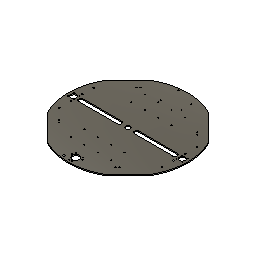
Baseplate-3mm (Autodesk Fusion 360 design; units mm, degrees)
Autodesk Fusion 360 part; units mm, degrees
sketch "Skizze1" plane through (0, 0, 0) normal (0, 0, 1) x (1, 0, 0)
  line L0 (0, 0) -> (-150, 0) construction
  line L1 (0, 0) -> (-24, 0) construction
  line L2 (-14, 0) -> (-130, 0) construction
  line L3 (0, 0) -> (95.4594, 95.4594) construction
  line L4 (0, 0) -> (-95.4594, 95.4594) construction
  line L5 (0, 0) -> (95.4594, -95.4594) construction
  line L6 (0, 0) -> (-95.4594, -95.4594) construction
  line L7 (-150, -16) -> (-142, -16) construction
  circle A0 centre (-142, -16) radius 2.1
  line L8 (-142, -16) -> (-142, -48) construction
  circle A1 centre (-142, -48) radius 2.1
  line L9 (-111.7229, 111.7229) -> (-78.1, 145.3458)
  line L10 (-111.7229, 111.7229) -> (-145.3458, 78.1)
  line L11 (95.4594, 95.4594) -> (111.7229, 111.7229) construction
  line L12 (111.7229, 111.7229) -> (145.3458, 78.1)
  line L13 (111.7229, 111.7229) -> (78.1, 145.3458)
  arc A2 (78.1, 145.3458) -> (-78.1, 145.3458) centre (0, 0) ccw
  line L14 (111.7229, -111.7229) -> (145.3458, -78.1)
  line L15 (111.7229, -111.7229) -> (78.1, -145.3458)
  arc A3 (145.3458, -78.1) -> (145.3458, 78.1) centre (0, 0) ccw
  line L16 (-111.7229, -111.7229) -> (-78.1, -145.3458)
  line L17 (-111.7229, -111.7229) -> (-145.3458, -78.1)
  arc A4 (-145.3458, 78.1) -> (-145.3458, -78.1) centre (0, 0) ccw
  arc A5 (-78.1, -145.3458) -> (78.1, -145.3458) centre (0, 0) ccw
  line L18 (-150, 16) -> (-142, 16) construction
  circle A6 centre (-142, 16) radius 2.1
  line L19 (-142, 16) -> (-142, 48) construction
  circle A7 centre (-142, 48) radius 2.1
  arc A8 (-24, -6.25) -> (-24, 6.25) centre (-24, 0) ccw
  arc A9 (-130, 6.25) -> (-130, -6.25) centre (-130, 0) ccw
  circle A10 centre (142, 48) radius 2.1
  circle A11 centre (142, -16) radius 2.1
  circle A12 centre (142, 16) radius 2.1
  line L20 (150, 0) -> (150, -16) construction
  line L21 (150, 0) -> (150, 16) construction
  line L22 (150, 16) -> (142, 16) construction
  line L23 (142, 16) -> (142, 48) construction
  line L24 (150, 0) -> (0, 0) construction
  line L25 (-0.0142, -0.0056) -> (23.9858, -0.0056) construction
  line L26 (14, -0.0076) -> (129.9927, -0.1231) construction
  arc A13 (129.9858, -6.3731) -> (129.9996, 6.1269) centre (129.9927, -0.1231) ccw
  line L27 (150, -16) -> (142, -16) construction
  line L28 (142, -16) -> (142, -48) construction
  circle A14 centre (142, -48) radius 2.1
  circle A15 centre (0, 0) radius 6.5
  line L29 (0, 0) -> (0, -144) construction
  circle A16 centre (0, -144) radius 10
  line L30 (0, -144) -> (-14, -144) construction
  line L31 (0, -144) -> (-10.6066, -133.3934) construction
  circle A17 centre (-10.6066, -133.3934) radius 1.5
  line L32 (0, -144) -> (-3.8823, -158.4889) construction
  circle A18 centre (-3.8823, -158.4889) radius 1.5
  line L33 (0, -144) -> (3.6235, -157.523) construction
  circle A19 centre (3.6235, -157.523) radius 1.5
  line L34 (0, -144) -> (9.8995, -134.1005) construction
  circle A20 centre (9.8995, -134.1005) radius 1.5
  line L35 (0, -144) -> (14.4889, -140.1177) construction
  circle A21 centre (14.4889, -140.1177) radius 1.5
  line L36 (0, 0) -> (0, -65) construction
  line L37 (0, -65) -> (18.5, -65) construction
  line L38 (18.5, -65) -> (18.5, -101.9) construction
  line L39 (18.5, -101.9) -> (-18.5, -101.9) construction
  line L40 (-18.5, -101.9) -> (-18.5, -65) construction
  circle A22 centre (-18.5, -65) radius 1.35
  circle A23 centre (-18.5, -101.9) radius 1.35
  circle A24 centre (18.5, -101.9) radius 1.35
  circle A25 centre (18.5, -65) radius 1.35
  line L41 (0, 0) -> (0, 65) construction
  line L42 (0, 65) -> (18.5, 65) construction
  line L43 (18.5, 65) -> (18.5, 101.9) construction
  line L44 (18.5, 101.9) -> (-18.5, 101.9) construction
  line L45 (-18.5, 101.9) -> (-18.5, 65) construction
  circle A26 centre (-18.5, 65) radius 1.35
  circle A27 centre (18.5, 65) radius 1.35
  circle A28 centre (18.5, 101.9) radius 1.35
  circle A29 centre (-18.5, 101.9) radius 1.35
  line L46 (18.5, -65) -> (55.4, -65) construction
  line L47 (18.5, -101.9) -> (55.4, -101.9) construction
  line L48 (-18.5, -65) -> (-55.4, -65) construction
  line L49 (-18.5, -101.9) -> (-55.4, -101.9) construction
  circle A30 centre (55.4, -65) radius 1.35
  circle A31 centre (55.4, -101.9) radius 1.35
  circle A32 centre (-55.4, -65) radius 1.35
  circle A33 centre (-55.4, -101.9) radius 1.35
  line L50 (18.5, 101.9) -> (55.4, 101.9) construction
  line L51 (18.5, 65) -> (55.4, 65) construction
  line L52 (-18.5, 65) -> (-55.4, 65) construction
  line L53 (-18.5, 101.9) -> (-55.4, 101.9) construction
  circle A34 centre (-55.4, 101.9) radius 1.35
  circle A35 centre (-55.4, 65) radius 1.35
  circle A36 centre (55.4, 65) radius 1.35
  circle A37 centre (55.4, 101.9) radius 1.35
  line L54 (-150, 16) -> (-150, 0) construction
  line L55 (-150, 0) -> (-150, -16) construction
  circle A38 centre (150, 0) radius 8.05
  circle A39 centre (-150, 0) radius 8.05
  line L56 (-150, 0) -> (-150, 8) construction
  line L57 (-150, 8) -> (-142, 8) construction
  line L58 (-142, 8) -> (-142, -8) construction
  line L59 (-142, -8) -> (-158, -8) construction
  line L60 (-158, -8) -> (-158, 8) construction
  circle A40 centre (-158, 8) radius 1.1
  circle A41 centre (-142, 8) radius 1.1
  circle A42 centre (-142, -8) radius 1.1
  circle A43 centre (-158, -8) radius 1.1
  line L61 (150, 0) -> (150, 8.0016) construction
  line L62 (150, 8.0016) -> (142, 8.0016) construction
  line L63 (142, 8.0016) -> (142, -7.9984) construction
  line L64 (142, -7.9984) -> (158, -7.9984) construction
  line L65 (158, -7.9984) -> (158, 8.0016) construction
  circle A44 centre (158, -7.9984) radius 1.1
  circle A45 centre (142, -7.9984) radius 1.1
  circle A46 centre (142, 8.0016) radius 1.1
  circle A47 centre (158, 8.0016) radius 1.1
  line L66 (0, 65) -> (0, 110) construction
  line L67 (0, 110) -> (-20, 110) construction
  circle A48 centre (-20, 110) radius 1.35
  line L68 (-20, 110) -> (32.1, 110.0005) construction
  line L69 (32.1, 110.0005) -> (32.1, 115.1005) construction
  circle A49 centre (32.1, 115.1005) radius 1.35
  line L70 (32.1, 115.1005) -> (32.1, 143.0005) construction
  circle A50 centre (32.1, 143.0005) radius 1.35
  line L71 (32.1, 143.0005) -> (32.1, 158.2005) construction
  line L72 (32.1, 158.2005) -> (-18.7, 158.2005) construction
  circle A51 centre (-18.7, 158.2005) radius 1.35
  line L73 (-130, 6.25) -> (-24, 6.25)
  line L74 (23.9879, 6.2444) -> (129.9996, 6.1269)
  line L75 (23.9858, -0.0056) -> (23.9858, -6.2556) construction
  line L76 (129.9858, -6.3731) -> (23.9858, -6.2556)
  line L77 (23.9858, -0.0056) -> (23.9858, 6.0001) construction
  line L78 (-24, 0) -> (-24, -6.25) construction
  line L79 (-24, -6.25) -> (-130, -6.25)
  arc A52 (23.9879, 6.2444) -> (23.9858, -6.2556) centre (23.9858, -0.0056) ccw
  line L80 (0, -144) -> (-13.523, -140.3765) construction
  line L81 (0, -144) -> (-12.5631, -144) construction
  circle A53 centre (-13.523, -140.3765) radius 1.5
  line L82 (-95.4594, -95.4594) -> (-107.1267, -83.7922) construction
  line L83 (-107.1267, -83.7922) -> (-112.8542, -78.0646) construction
  circle A54 centre (-107.1267, -83.7922) radius 1.5
  circle A55 centre (-112.8542, -78.0646) radius 1.5
  line L84 (-95.4594, 95.4594) -> (-83.7922, 107.1267) construction
  line L85 (-83.7922, 107.1267) -> (-78.0646, 112.8542) construction
  line L86 (-83.7922, 107.1267) -> (-69.8987, 107.1267) construction
  circle A56 centre (-83.7922, 107.1267) radius 1.5
  circle A57 centre (-78.0646, 112.8542) radius 1.5
  line L87 (95.4594, 95.4594) -> (107.1267, 83.7922) construction
  line L88 (107.1267, 83.7922) -> (112.8542, 78.0646) construction
  circle A58 centre (107.1267, 83.7922) radius 1.5
  circle A59 centre (112.8542, 78.0646) radius 1.5
  line L89 (95.4594, -95.4594) -> (83.7922, -107.1267) construction
  line L90 (83.7922, -107.1267) -> (78.0646, -112.8542) construction
  circle A60 centre (83.7922, -107.1267) radius 1.5
  circle A61 centre (78.0646, -112.8542) radius 1.5
  line L91 (0, -144) -> (-20.7846, -156) construction
  circle A62 centre (-20.7846, -156) radius 2.65
  dimension "d144" = 4.2
  dimension "d148" = 4.2
  dimension "d185" = 4.2
  dimension "d187" = 4.2
  dimension "d306" = 12.5
  dimension "d309" = 12.5
  dimension "d333" = 4.2
  dimension "d335" = 4.2
  dimension "d338" = 4.2
  dimension "d371" = 12.5
  dimension "d383" = 4.2
  dimension "d386" = 13
  dimension "d390" = 20
  dimension "d400" = 3
  dimension "d402" = 3
  dimension "d405" = 3
  dimension "d408" = 3
  dimension "d411" = 3
  dimension "d419" = 2.7
  dimension "d420" = 2.7
  dimension "d421" = 2.7
  dimension "d422" = 2.7
  dimension "d428" = 2.7
  dimension "d429" = 2.7
  dimension "d430" = 2.7
  dimension "d431" = 2.7
  dimension "d438" = 2.7
  dimension "d439" = 2.7
  dimension "d440" = 2.7
  dimension "d441" = 2.7
  dimension "d446" = 2.7
  dimension "d447" = 2.7
  dimension "d448" = 2.7
  dimension "d449" = 2.7
  dimension "d456" = 16.1
  dimension "d457" = 16.1
  dimension "d463" = 2.2
  dimension "d464" = 2.2
  dimension "d465" = 2.2
  dimension "d466" = 2.2
  dimension "d473" = 2.2
  dimension "d474" = 2.2
  dimension "d475" = 2.2
  dimension "d476" = 2.2
  dimension "d483" = 45
  dimension "d484" = 20
  dimension "d485" = 2.7
  dimension "d488" = 2.7
  dimension "d490" = 5.1
  dimension "d491" = 27.9
  dimension "d492" = 52.1
  dimension "d493" = 2.7
  dimension "d494" = 15.2
  dimension "d495" = 50.8
  dimension "d497" = 2.7
  dimension "d505" = 144
  dimension "d506" = 135
  dimension "d507" = 45
  dimension "d508" = 165
  dimension "d509" = 105
  dimension "d510" = 75
  dimension "d511" = 14
  dimension "d512" = 15
  dimension "d513" = 14
  dimension "d514" = 15
  dimension "d515" = 14
  dimension "d516" = 15
  dimension "d522" = 106
  dimension "d526" = 106
  dimension "d527" = 12.5
  dimension "d530" = 150
  dimension "d531" = 150
  dimension "d532" = 8
  dimension "d533" = 16
  dimension "d534" = 16
  dimension "d535" = 16
  dimension "d536" = 16
  dimension "d537" = 16
  dimension "d538" = 8
  dimension "d539" = 32
  dimension "d540" = 32
  dimension "d541" = 8
  dimension "d542" = 32
  dimension "d543" = 8
  dimension "d544" = 16
  dimension "d545" = 16
  dimension "d546" = 16
  dimension "d547" = 16
  dimension "d548" = 8
  dimension "d549" = 16
  dimension "d550" = 8
  dimension "d551" = 32
  dimension "d552" = 135
  dimension "d553" = 135
  dimension "d554" = 135
  dimension "d555" = 135
  dimension "d564" = 36.9
  dimension "d565" = 36.9
  dimension "d566" = 36.9
  dimension "d567" = 37
  dimension "d568" = 18.5
  dimension "d569" = 36.9
  dimension "d570" = 36.9
  dimension "d571" = 36.9
  dimension "d572" = 65
  dimension "d575" = 47.55
  dimension "d576" = 47.55
  dimension "d577" = 165
  dimension "d578" = 47.55
  dimension "d579" = 47.55
  dimension "d580" = 165
  dimension "d581" = 47.55
  dimension "d582" = 47.55
  dimension "d583" = 165
  dimension "d584" = 47.55
  dimension "d585" = 47.55
  dimension "d586" = 165
  dimension "d589" = 15
  dimension "d590" = 14
  dimension "d591" = 3
  dimension "d594" = 36.9
  dimension "d595" = 36.9
  dimension "d596" = 36.9
  dimension "d597" = 37
  dimension "d598" = 18.5
  dimension "d599" = 36.9
  dimension "d600" = 36.9
  dimension "d601" = 36.9
  dimension "d604" = 16.5
  dimension "d605" = 8.1
  dimension "d606" = 3
  dimension "d607" = 3
  dimension "d608" = 16.5
  dimension "d609" = 45
  dimension "d610" = 8.1
  dimension "d611" = 3
  dimension "d612" = 3
  dimension "d613" = 16.5
  dimension "d614" = 8.1
  dimension "d615" = 3
  dimension "d616" = 3
  dimension "d617" = 16.5
  dimension "d618" = 8.1
  dimension "d619" = 3
  dimension "d620" = 3
  dimension "d623" = 24
  dimension "d624" = 24
  dimension "d631" = 24
  dimension "d632" = 45
  dimension "d633" = 5.3
  constraint coincident L0.start L1.start
  constraint parallel L0 L1
  constraint parallel L0 L2
  constraint coincident L7.end A0.centre
  constraint perpendicular L7 L8
  constraint coincident L8.end A1.centre
  constraint concentric A2 A4
  constraint concentric A3 A4
  constraint concentric A4 A5
  constraint coincident L18.end A6.centre
  constraint perpendicular L18 L19
  constraint coincident L19.end A7.centre
  constraint coincident L1.end A8.centre
  constraint coincident L2.end A9.centre
  constraint perpendicular L21 L22
  constraint coincident A12.centre L22.end
  constraint perpendicular L22 L23
  constraint coincident A10.centre L23.end
  constraint perpendicular L21 L24
  constraint parallel L24 L25
  constraint coincident L26.end A13.centre
  constraint perpendicular L20 L24
  constraint coincident A11.centre L27.end
  constraint perpendicular L27 L28
  constraint coincident L28.end A14.centre
  constraint concentric A5 A15
  constraint vertical L29
  constraint coincident L29.end A16.centre
  constraint perpendicular L29 L30
  constraint coincident L31.end A17.centre
  constraint coincident L32.end A18.centre
  constraint coincident L33.end A19.centre
  constraint coincident L34.end A20.centre
  constraint coincident L35.end A21.centre
  constraint perpendicular L25 L36
  constraint perpendicular L29 L37
  constraint perpendicular L37 L38
  constraint perpendicular L38 L39
  constraint perpendicular L39 L40
  constraint coincident L40.end A22.centre
  constraint coincident L39.end L40.start
  constraint coincident L38.end L39.start
  constraint coincident L37.end L38.start
  constraint perpendicular L24 L41
  constraint perpendicular L41 L42
  constraint perpendicular L42 L43
  constraint perpendicular L43 L44
  constraint perpendicular L44 L45
  constraint coincident L45.end A26.centre
  constraint coincident L42.end L43.start
  constraint coincident L43.end L44.start
  constraint coincident L44.end L45.start
  constraint perpendicular L38 L46
  constraint perpendicular L38 L47
  constraint perpendicular L40 L48
  constraint perpendicular L40 L49
  constraint coincident L46.end A30.centre
  constraint coincident L47.end A31.centre
  constraint coincident L48.end A32.centre
  constraint coincident L49.end A33.centre
  constraint perpendicular L43 L50
  constraint perpendicular L43 L51
  constraint perpendicular L45 L52
  constraint perpendicular L45 L53
  constraint coincident L53.end A34.centre
  constraint coincident L52.end A35.centre
  constraint coincident L51.end A36.centre
  constraint coincident L50.end A37.centre
  constraint perpendicular L0 L54
  constraint perpendicular L7 L55
  constraint perpendicular L18 L54
  constraint perpendicular L0 L55
  constraint perpendicular L20 L27
  constraint coincident L20.start L21.start
  constraint coincident L0.end L54.end
  constraint perpendicular L0 L56
  constraint perpendicular L56 L57
  constraint perpendicular L0 L58
  constraint perpendicular L55 L59
  constraint perpendicular L59 L60
  constraint coincident L60.end A40.centre
  constraint coincident L57.end L58.start
  constraint coincident L58.end L59.start
  constraint coincident L59.end L60.start
  constraint perpendicular L24 L61
  constraint perpendicular L61 L62
  constraint perpendicular L62 L63
  constraint perpendicular L20 L64
  constraint perpendicular L64 L65
  constraint coincident L64.end L65.start
  constraint coincident L63.end L64.start
  constraint coincident L62.end L63.start
  constraint coincident L65.end A47.centre
  constraint perpendicular L44 L66
  constraint perpendicular L66 L67
  constraint coincident L67.end A48.centre
  constraint perpendicular L68 L69
  constraint coincident L69.end A49.centre
  constraint vertical L41
  constraint vertical L70
  constraint coincident L70.end A50.centre
  constraint parallel L70 L71
  constraint perpendicular L71 L72
  constraint coincident L72.end A51.centre
  constraint horizontal L73
  constraint tangent A13 L74
  constraint perpendicular L24 L75
  constraint perpendicular L24 L77
  constraint perpendicular L1 L78
  constraint coincident L25.end L75.start
  constraint horizontal L0
  constraint horizontal L81
  constraint coincident L80.end A53.centre
  constraint perpendicular L6 L82
  constraint parallel L82 L83
  constraint coincident L82.end L83.start
  constraint coincident L83.end A55.centre
  constraint perpendicular L4 L84
  constraint horizontal L86
  constraint coincident L84.end L85.start
  constraint coincident L85.end A57.centre
  constraint perpendicular L3 L87
  constraint perpendicular L3 L88
  constraint coincident L87.end L88.start
  constraint coincident L88.end A59.centre
  constraint perpendicular L5 L89
  constraint parallel L89 L90
  constraint coincident L89.end L90.start
  constraint coincident L90.end A61.centre
  constraint tangent A13 L76
  constraint tangent A9 L73
  constraint tangent A8 L73
  constraint tangent A9 L79
  constraint coincident L91.end A62.centre
  measures "d144" diameter of A0
  measures "d148" diameter of A1
  measures "d185" diameter of A6
  measures "d187" diameter of A7
  measures "d306" diameter of A8
  measures "d309" diameter of A9
  measures "d333" diameter of A12
  measures "d335" diameter of A10
  measures "d338" diameter of A11
  measures "d371" diameter of A13
  measures "d383" diameter of A14
  measures "d386" diameter of A15
  measures "d390" diameter of A16
  measures "d400" diameter of A17
  measures "d402" diameter of A18
  measures "d405" diameter of A19
  measures "d408" diameter of A20
  measures "d411" diameter of A21
  measures "d419" diameter of A22
  measures "d420" diameter of A23
  measures "d421" diameter of A24
  measures "d422" diameter of A25
  measures "d428" diameter of A26
  measures "d429" diameter of A27
  measures "d430" diameter of A28
  measures "d431" diameter of A29
  measures "d438" diameter of A30
  measures "d439" diameter of A31
  measures "d440" diameter of A32
  measures "d441" diameter of A33
  measures "d446" diameter of A34
  measures "d447" diameter of A35
  measures "d448" diameter of A36
  measures "d449" diameter of A37
  measures "d456" diameter of A38
  measures "d457" diameter of A39
  measures "d463" diameter of A40
  measures "d464" diameter of A41
  measures "d465" diameter of A42
  measures "d466" diameter of A43
  measures "d473" diameter of A44
  measures "d474" diameter of A45
  measures "d475" diameter of A46
  measures "d476" diameter of A47
  measures "d483" distance of L41.end L66.end
  measures "d484" distance of L66.end L67.end
  measures "d485" diameter of A48
  measures "d488" diameter of A49
  measures "d490" vertical distance of L68.end L69.end
  measures "d491" distance of L69.end L70.end
  measures "d492" horizontal distance of L67.end L68.end
  measures "d493" diameter of A50
  measures "d494" distance of L70.end L71.end
  measures "d495" distance of L71.end L72.end
  measures "d497" diameter of A51
  measures "d505" distance of L0.start L29.end
  measures "d506" angle of L30 L34
  measures "d507" angle of L30 L31
  measures "d508" angle of L30 L35
  measures "d509" angle of L30 L33
  measures "d510" angle of L30 L32
  measures "d511" distance of L29.end L34.end
  measures "d512" distance of L29.end L35.end
  measures "d513" distance of L29.end L33.end
  measures "d514" distance of L29.end L32.end
  measures "d515" distance of L29.end L30.end
  measures "d516" distance of L29.end L31.end
  measures "d522" distance of A13.start L75.end
  measures "d526" distance of A9.end A8.start
  measures "d527" diameter of A52
  measures "d530" distance of L0.start L0.end
  measures "d531" distance of L0.start L20.start
  measures "d532" distance of L56.end L57.end
  measures "d533" distance of L57.end L58.end
  measures "d534" distance of L58.end L59.end
  measures "d535" distance of L59.end L60.end
  measures "d536" distance of L0.end L18.start
  measures "d537" distance of L0.end L7.start
  measures "d538" distance of L7.start L7.end
  measures "d539" distance of L7.end L8.end
  measures "d540" distance of L18.end L19.end
  measures "d541" distance of L18.start L18.end
  measures "d542" distance of A12.centre A10.centre
  measures "d543" distance of L21.end A12.centre
  measures "d544" distance of L20.start L21.end
  measures "d545" distance of L64.end L65.end
  measures "d546" distance of L63.end L64.end
  measures "d547" distance of L62.end L63.end
  measures "d548" distance of L61.end L62.end
  measures "d549" distance of L20.start L20.end
  measures "d550" distance of L20.end A11.centre
  measures "d551" distance of A11.centre L28.end
  measures "d552" distance of L0.start L4.end
  measures "d553" distance of L0.start L3.end
  measures "d554" distance of L0.start L6.end
  measures "d555" distance of L0.start L5.end
  measures "d564" distance of L43.end L50.end
  measures "d565" distance of L42.end L51.end
  measures "d566" distance of L42.end L43.end
  measures "d567" distance of L43.end L44.end
  measures "d568" distance of L41.end L42.end
  measures "d569" distance of L44.end L45.end
  measures "d570" distance of L44.end L53.end
  measures "d571" distance of L45.end L52.end
  measures "d572" distance of L0.start L41.end
  measures "d575" distance of L16.start L16.end
  measures "d576" distance of L16.start L17.end
  measures "d577" radius of A5
  measures "d578" distance of L14.start L15.end
  measures "d579" distance of L14.start L14.end
  measures "d580" radius of A3
  measures "d581" distance of L11.end L12.end
  measures "d582" distance of L11.end L13.end
  measures "d583" radius of A2
  measures "d584" distance of L9.start L9.end
  measures "d585" distance of L9.start L10.end
  measures "d586" radius of A4
  measures "d589" angle of L80 L81
  measures "d590" distance of L29.end L80.end
  measures "d591" diameter of A53
  measures "d594" distance of L40.end L48.end
  measures "d595" distance of L39.end L49.end
  measures "d596" distance of L39.end L40.end
  measures "d597" distance of L38.end L39.end
  measures "d598" distance of L36.end L37.end
  measures "d599" distance of L37.end L46.end
  measures "d600" distance of L38.end L47.end
  measures "d601" distance of L37.end L38.end
  measures "d604" distance of L6.end L82.end
  measures "d605" distance of L82.end L83.end
  measures "d606" diameter of A54
  measures "d607" diameter of A55
  measures "d608" distance of L4.end L84.end
  measures "d609" angle of L85 L86
  measures "d610" distance of L84.end L85.end
  measures "d611" diameter of A56
  measures "d612" diameter of A57
  measures "d613" distance of L3.end L87.end
  measures "d614" distance of L87.end L88.end
  measures "d615" diameter of A58
  measures "d616" diameter of A59
  measures "d617" distance of L5.end L89.end
  measures "d618" distance of L89.end L90.end
  measures "d619" diameter of A60
  measures "d620" diameter of A61
  measures "d623" distance of L0.start L1.end
  measures "d624" distance of L25.start L25.end
  measures "d631" distance of L29.end L91.end
  measures "d632" angle of L80 L91
  measures "d633" diameter of A62
extrude "Extrusion23" add sketch "Skizze1" along normal blind 3
extrude "Extrusion19" [suppressed]
extrude "Extrusion20" [suppressed]
extrude "Extrusion21" [suppressed]
extrude "Extrusion17" [suppressed]
extrude "Extrusion16" [suppressed]
extrude "Extrusion15" [suppressed]
extrude "Extrusion14" [suppressed]
extrude "Extrusion13" [suppressed]
extrude "Extrusion12" [suppressed]
extrude "Extrusion10" [suppressed]
